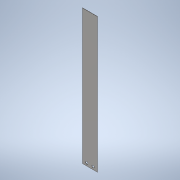
# Autodesk Inventor part: tape
Saved by Autodesk Inventor 2022 (Build 260153000, 153)
## iProperties
Created: 2022-04-25
Part Number: tape
Material: Stainless Steel
Document SubType Name: Modeling
Designer: Bowen
Density: 8 g/cm^3
Appearance: Semi-Polished
Author: Bowen
Autodesk Inventor part; units mm, degrees
ref_plane "YZ Plane" through (0, 0, 0) normal (1, 0, 0) x (0, 1, 0)
ref_plane "XZ Plane" through (0, 0, 0) normal (0, 1, 0) x (-1, 0, 0)
ref_plane "XY Plane" through (0, 0, 0) normal (0, 0, 1) x (1, 0, 0)
sketch "Sketch1" plane through (0, 0, 0) normal (0, 0, 1) x (1, 0, 0)
  line L0 (-9.525, -125) -> (9.525, -125)
  line L1 (9.525, -125) -> (9.525, 125)
  line L2 (9.525, 125) -> (-9.525, 125)
  line L3 (-9.525, 125) -> (-9.525, -125)
  point P0 (0, 0)
  point P1 (0, -125)
  point P2 (9.525, 0)
  dimension "d0" = 19.05
  dimension "d1" = 250
  constraints: 8 end point, 2 midpoint, 2 parallel, 1 horizontal, 1 horizontal alignment, 1 perpendicular, 1 vertical alignment
  measures "d0" distance of L2.end L1.end
  measures "d1" distance of L0.end L1.end
extrude "Extrusion1" add sketch "Sketch1" along normal blind 0.25
sketch "Sketch3" plane through (0, 0, 0.25) normal (0, 0, 1) x (1, 0, 0)
  line L0 (-9.525, 125) -> (-9.525, -125) projected
  line L1 (9.525, -125) -> (9.525, 125) projected
  line L2 (9.525, -125) -> (9.525, -122.36)
  line L3 (-9.525, -122.36) -> (-9.525, -125)
  line L4 (0, -125) -> (-4, -125) construction
  line L5 (-4, -125) -> (-4, -121.5) construction
  point P0 (0, 0)
  dimension "d18" = 4
  dimension "d19" = 3.5
  constraints: 8 end point, 1 parallel, 1 point on line
  measures "d18" distance of L4.start L4.end
  measures "d19" distance of L4.end L5.end
hole "Hole2" at (-4, -121.5, 0.25) direction (0, 0, -1) diameter 3 end through all
mirror "Mirror1" about plane through (0, 0, 0) normal (1, 0, 0) of "Hole2"
sketch "Sketch4" plane through (0, 0, 0.25) normal (0, 0, 1) x (1, 0, 0)
  line L0 (-9.525, 125) -> (-9.525, -125) projected
  line L1 (9.525, -125) -> (9.525, 125) projected
  line L2 (-9.525, -125) -> (9.525, -125)
  line L3 (9.525, -125) -> (9.525, 46.45)
  line L4 (9.525, 46.45) -> (-9.525, 46.45)
  line L5 (-9.525, 46.45) -> (-9.525, -125)
  point P0 (0, 0)
  dimension "d27" = 171.45
  constraints: 8 end point, 2 parallel, 1 horizontal, 1 perpendicular, 1 point on line
  measures "d27" distance of L3.end L2.end
extrude "Extrusion2" cut sketch "Sketch4" against normal blind 10 keep common part
body "Solid1"
